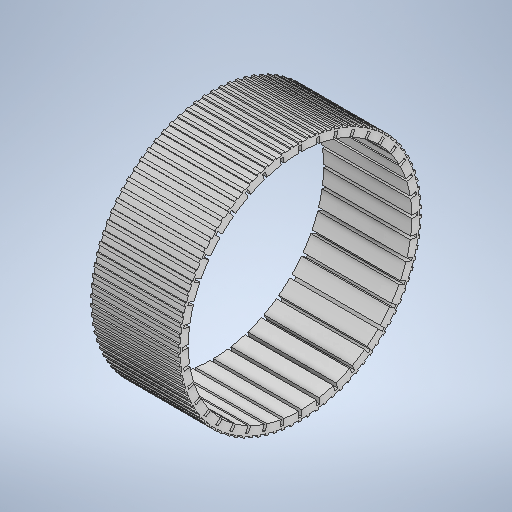
# Autodesk Inventor part: pneu
Saved by Autodesk Inventor 2026.2 (Build 302298010, 298A)
## iProperties
Created: 2026-05-13
Part Number: pneu
Material: Générique
Document SubType Name: Modeling
Designer: Genon
Density: 1 g/cm^3
Appearance: Par défaut
Author: Genon
Autodesk Inventor part; units mm, degrees
ref_plane "YZ Plane" through (0, 0, 0) normal (1, 0, 0) x (0, 1, 0)
ref_plane "XZ Plane" through (0, 0, 0) normal (0, 1, 0) x (-1, 0, 0)
ref_plane "XY Plane" through (0, 0, 0) normal (0, 0, 1) x (1, 0, 0)
sketch "Esquisse1" plane through (0, 0, 0) normal (1, 0, 0) x (0, 1, 0)
  circle A0 centre (0, 0) radius 40
  circle A1 centre (0, 0) radius 38
  circle A2 centre (0, 0) radius 40.75
  dimension "d0" = 80
  dimension "d1" = 76
  dimension "d9" = 81.5
  constraints: 3 centre point, 3 coincident
  measures "d0" diameter of A0
  measures "d1" diameter of A1
  measures "d9" diameter of A2
extrude "Extrusion1" add sketch "Esquisse1" along normal blind 30 contours A0 | A2
sketch "Esquisse2" plane through (30, 0, 0) normal (1, 0, 0) x (0, 0, -1)
  circle A0 centre (0, 0) radius 38 projected
  line L0 (0, 38) -> (0, 40)
  line L1 (0, 40) -> (0.5, 40)
  line L2 (0.5, 40) -> (0.5, 37.9967)
  line L3 (0, 40) -> (-0.5, 40)
  line L4 (-0.5, 40) -> (-0.4872, 37.9969)
  dimension "d4" = 2
  dimension "d5" = 0.5
  dimension "d6" = 0.5
  constraints: 10 end point, 3 point on circle, 2 perpendicular, 1 point on line, 1 vertical
  measures "d4" distance of L0.start L0.end
  measures "d5" distance of L0.end L1.end
  measures "d6" distance of L0.end L3.end
extrude "Extrusion2" cut sketch "Esquisse2" against normal up to surface (30 mm away) contours A0 L0 L1 L2 | L4 L3 L0 A0
pattern_circular "Réseau circulaire1" count 40 over 360 about axis through (-10, 0, 0) along (1, 0, 0) of "Extrusion2"
sketch "Esquisse3" plane through (30, 0, 0) normal (1, 0, 0) x (0, 0, -1)
  circle A0 centre (0, 0) radius 40.75 projected
  line L0 (0, 40.75) -> (0, 41.25)
  line L1 (0, 41.25) -> (0.5, 41.25)
  line L2 (0, 41.25) -> (-0.5, 41.25)
  line L3 (-0.5, 41.25) -> (-0.5, 40.7469)
  line L4 (0.5, 41.25) -> (0.5, 40.7469)
  dimension "d13" = 0.5
  dimension "d14" = 0.5
  dimension "d15" = 0.5
  constraints: 10 end point, 3 point on circle, 2 perpendicular, 2 vertical, 1 horizontal
  measures "d13" distance of L0.start L0.end
  measures "d14" distance of L0.end L1.end
  measures "d15" distance of L0.end L2.end
extrude "Extrusion3" add sketch "Esquisse3" against normal blind 30 contours A0 L0 L1 L4 | L3 L2 L0 A0
pattern_circular "Réseau circulaire2" count 90 over 360 about axis through (-10, 0, 0) along (1, 0, 0) of "Extrusion3"
